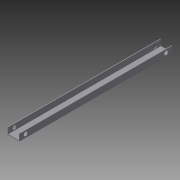
# Autodesk Inventor part: U-Channel
Saved by Autodesk Inventor 2013 (Build 170138000, 138)
## iProperties
Created: 2014-01-30
Part Number: U-Channel
Material: Generic
Document SubType Name: Modeling
Designer: nojessen
Density: 1 g/cm^3
Author: nojessen
Autodesk Inventor part; units mm, degrees
ref_plane "YZ Plane" through (0, 0, 0) normal (1, 0, 0) x (0, 1, 0)
ref_plane "XZ Plane" through (0, 0, 0) normal (0, 1, 0) x (-1, 0, 0)
ref_plane "XY Plane" through (0, 0, 0) normal (0, 0, 1) x (1, 0, 0)
sketch "Sketch1" plane through (0, 0, 0) normal (0, 0, 1) x (1, 0, 0)
  line L0 (0, 13.97) -> (0, 0)
  line L1 (0, 0) -> (24.8666, 0)
  line L2 (24.8666, 0) -> (24.8666, 13.97)
  line L3 (23.5966, 13.97) -> (23.5966, 1.27)
  line L4 (23.5966, 1.27) -> (1.27, 1.27)
  line L5 (1.27, 1.27) -> (1.27, 13.97)
  line L6 (24.8666, 13.97) -> (23.5966, 13.97)
  line L7 (1.27, 13.97) -> (0, 13.97)
  dimension "d0" = 24.8666
  dimension "d2" = 13.97
  dimension "d3" = 1.27
  dimension "d4" = 1.27
  dimension "d5" = 1.27
  constraints: 16 end point, 4 parallel, 2 horizontal, 2 perpendicular
  measures "d0" distance of L2.end L0.start
  measures "d2" distance of L1.end L2.end
  measures "d3" distance between parallel lines of L0 L5
  measures "d4" distance between parallel lines of L1 L4
  measures "d5" distance between parallel lines of L2 L3
extrude "Extrusion1" add sketch "Sketch1" along normal blind 317.5
sketch "Sketch2" plane through (24.8666, 0, 0) normal (1, 0, 0) x (0, 0, -1)
  line L0 (0, 13.97) -> (0, 0) projected
  line L1 (-317.5, 0) -> (-317.5, 13.97) projected
  circle A0 centre (-304.8, 6.985) radius 4.0005
  circle A1 centre (-12.7, 6.985) radius 4.0005
  dimension "d8" = 8.001
  dimension "d9" = 8.001
  dimension "d10" = 12.7
  dimension "d11" = 12.7
  constraints: 2 centre point
  measures "d8" diameter of A0
  measures "d9" diameter of A1
  measures "d10" distance from line of L1 A0.centre
  measures "d11" distance from line of L0 A1.centre
extrude "Extrusion2" cut sketch "Sketch2" against normal blind 317.5 contours A1
sketch "Sketch3" plane through (24.8666, 0, 0) normal (1, 0, 0) x (0, 0, -1)
  line L0 (-317.5, 0) -> (-317.5, 13.97) projected
  circle A0 centre (-304.8, 6.985) radius 4.0005
  dimension "d14" = 8.001
  dimension "d15" = 12.7
  constraints: 1 centre point
  measures "d14" diameter of A0
  measures "d15" distance from line of L0 A0.centre
extrude "Extrusion3" cut sketch "Sketch3" against normal blind 317.5
body "Solid1"
